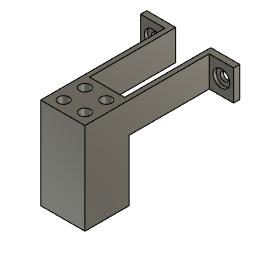
tube_holder (Autodesk Fusion 360 design; units mm, degrees)
Autodesk Fusion 360 part; units mm, degrees
sketch "Sketch1" plane through (0, 0, 0) normal (0, 0, 1) x (1, 0, 0) in component "Halterung"
  line L0 (0, 0) -> (29, 0)
  line L1 (29, 0) -> (29, 29)
  line L2 (29, 29) -> (0, 29)
  line L3 (0, 29) -> (0, 0)
  circle A0 centre (7.5, 7.5) radius 3.5
  circle A1 centre (21.5, 7.5) radius 3.5
  circle A2 centre (7.5, 21.5) radius 3.5
  circle A3 centre (21.5, 21.5) radius 3.5
  dimension "d1" = 7
  dimension "d3" = 4
  dimension "d6" = 7
  dimension "d7" = 4
  dimension "d8" = 7
  dimension "d9" = 4
  dimension "d10" = 4
  dimension "d15" = 35
  constraint horizontal L0
  constraint vertical L1
  constraint horizontal L2
  constraint vertical L3
  constraint coincident L0.start L3.end
  constraint equal A0 A2
  constraint equal A0 A3
  constraint equal A0 A1
  constraint horizontal A0.centre A1.centre
  constraint vertical A0.centre A2.centre
  constraint horizontal A2.centre A3.centre
  constraint vertical A1.centre A3.centre
  measures "d1" diameter of A0
  measures "d3" distance of L0 A0
  measures "d6" distance of A0 A2
  measures "d7" distance of L2 A2
  measures "d8" distance of A2 A3
  measures "d9" distance of L1 A3
  measures "d10" distance of L3 A2
extrude "Extrude1" add sketch "Sketch1" along normal blind 60 in component "Halterung"
sketch "Sketch2" plane through (0, 29, 0) normal (0, 1, 0) x (-1, 0, 0) in component "Halterung"
  line L0 (-29, 0) -> (0, 0)
  line L1 (0, 0) -> (0, 60)
  line L2 (0, 60) -> (-29, 60)
  line L3 (-29, 60) -> (-29, 0)
  line L4 (-29, 60) -> (-26, 60)
  line L5 (-26, 60) -> (-26, 40)
  line L6 (-26, 40) -> (-29, 40)
  line L7 (-29, 40) -> (-29, 60)
  line L8 (-14.5, 60) -> (-14.5, 0) construction
  line L9 (-3, 60) -> (-3, 40)
  line L10 (0, 60) -> (-3, 60)
  line L11 (0, 40) -> (0, 60)
  line L12 (-3, 40) -> (0, 40)
  dimension "d13" = 3
  dimension "d14" = 20
  constraint horizontal L4
  constraint vertical L5
  constraint horizontal L6
  constraint vertical L7
  constraint coincident L2.end L3.start
  constraint midpoint L2 L8.start
  constraint midpoint L0 L8.end
  constraint symmetric L2.end L8 L1.end
  constraint symmetric L4.end L8 L9.start
  constraint symmetric L5.end L8 L9.end
  constraint symmetric L6.end L8 L11.start
  measures "d13" distance of L2.end L4.end
  measures "d14" distance of L2.end L6.end
extrude "Extrude2" add sketch "Sketch2" along normal blind 56.5 contours L2 L3 L4 L5 L6 L7 | L1 L2 L9 L10 L11 L12 in component "Halterung"
sketch "Sketch3" plane through (29, 0, 0) normal (1, 0, 0) x (0, 1, 0) in component "Halterung"
  line L0 (0, 0) -> (29, 0)
  line L1 (29, 0) -> (29, 40)
  line L2 (29, 40) -> (85.5, 40)
  line L3 (85.5, 40) -> (85.5, 60)
  line L4 (85.5, 60) -> (0, 60)
  line L5 (0, 60) -> (0, 0)
  line L6 (85.5, 60) -> (81.5, 60)
  line L7 (81.5, 60) -> (81.5, 40)
  line L8 (81.5, 40) -> (85.5, 40)
  line L9 (85.5, 40) -> (85.5, 60)
  dimension "d18" = 4
  constraint horizontal L6
  constraint vertical L7
  constraint horizontal L8
  constraint vertical L9
  constraint coincident L2 L7.end
  constraint coincident L3.end L4.start
  measures "d18" distance of L3.end L6.end
extrude "Extrude3" add sketch "Sketch3" along normal blind 16 contours L2 L3 L4 L6 L7 L8 L9 in component "Halterung"
extrude "Extrude4" add sketch "Sketch3" against normal blind 16 from surface at -29 contours L2 L3 L4 L6 L7 L8 L9 in component "Halterung"
sketch "Sketch4" plane through (0, 81.5, 0) normal (0, -1, 0) x (1, 0, 0) in component "Halterung"
  line L0 (29, 60) -> (29, 40)
  line L1 (29, 40) -> (45, 40)
  line L2 (45, 40) -> (45, 60)
  line L3 (45, 60) -> (29, 60)
  circle A0 centre (37, 50) radius 5.5
  line L4 (45, 50) -> (29, 50) construction
  line L5 (37, 60) -> (37, 40) construction
  line L6 (14.5, 0) -> (14.5, 60) construction
  line L7 (0, 60) -> (29, 60)
  line L8 (0, 0) -> (29, 0)
  circle A1 centre (37, 50) radius 2.75
  circle A2 centre (-8, 50) radius 5.5
  circle A3 centre (-8, 50) radius 2.75
  point P0 (37, 50)
  dimension "d24" = 11
  dimension "d25" = 5.5
  constraint midpoint L2 L4.start
  constraint midpoint L0 L4.end
  constraint midpoint L3 L5.start
  constraint midpoint L1 L5.end
  constraint midpoint L5 P0
  constraint midpoint P0 L4
  constraint vertical L6
  constraint midpoint L6.end L7
  constraint coincident L6.start L8
  constraint coincident P0 A0.centre
  constraint symmetric A0 L6 A2
  constraint symmetric L6 A1 A3
  measures "d24" diameter of A0
  measures "d25" diameter of A1
extrude "Extrude5" cut sketch "Sketch4" against normal up to surface (4 mm away) contours A1 | A3 in component "Halterung"
extrude "Extrude6" cut sketch "Sketch4" against normal blind 2 contours A0 | A2 in component "Halterung"
sketch "Sketch1 (2)" plane through (0, 0, 0) normal (0, 0, -1) x (1, 0, 0)
  line L0 (0, 0) -> (0, -29)
  line L1 (0, -29) -> (29, -29)
  line L2 (29, -29) -> (29, 0)
  line L3 (29, 0) -> (0, 0)
  circle A0 centre (7.5, -7.5) radius 2.9
  circle A1 centre (21.5, -7.5) radius 2.9
  circle A2 centre (7.5, -21.5) radius 2.9
  circle A3 centre (21.5, -21.5) radius 2.9
  circle A4 centre (21.5, -21.5) radius 3.5
  circle A5 centre (7.5, -21.5) radius 3.5
  circle A6 centre (21.5, -7.5) radius 3.5
  circle A7 centre (7.5, -7.5) radius 3.5
  dimension "d52" = 5.8
  constraint concentric A2 A5
  constraint concentric A3 A4
  constraint concentric A1 A6
  constraint concentric A0 A7
  constraint equal A0 A2
  constraint equal A0 A1
  constraint equal A1 A3
  measures "d52" diameter of A2
extrude "Extrude9" add sketch "Sketch1 (2)" against normal blind 5 contours A4 | A5 | A6 | A7 in component "Halterung"
chamfer "Chamfer2" distance 3 angle 45 4 edges at (4.7963, 20.4513, 0) (18.7963, 20.4513, 0) (18.7963, 6.4513, 0) (4.7963, 6.4513, 0) in component "Halterung"
component "Halterung" placed x (1, 0, 0) y (0, 1, 0) z (0, 0, 1) at (0, 0, 0)
